VIHALS Motor Side Wire Holder (Autodesk Fusion 360 design; units mm, degrees)
Autodesk Fusion 360 part; units mm, degrees
sketch "Sketch1" plane through (0, 0, 0) normal (0, 0, 1) x (1, 0, 0)
  line L0 (-12.5, 10) -> (12.5, 10)
  line L1 (12.5, 10) -> (12.5, -10)
  line L2 (12.5, -10) -> (-12.5, -10)
  line L3 (-12.5, -10) -> (-12.5, 10)
  dimension "d1" = 25
  dimension "d2" = 12.5
  dimension "d3" = 20
  dimension "d4" = 10
  constraint horizontal L0
  constraint vertical L1
  constraint horizontal L2
  constraint vertical L3
  measures "d1" distance of L1 L3
  measures "d2" distance of origin L1
  measures "d3" distance of L0 L2
  measures "d4" distance of origin L0
extrude "Extrude1" add sketch "Sketch1" along normal blind 2
sketch "Sketch2" plane through (0, 0, 2) normal (0, 0, 1) x (-1, 0, 0)
  line L0 (12.5, 10) -> (-12.5, 10)
  line L1 (-12.5, 10) -> (-12.5, -10)
  line L2 (-12.5, -10) -> (12.5, -10)
  line L3 (12.5, -10) -> (12.5, 10)
  line L4 (12.5, 10) -> (14.5, 10)
  line L5 (14.5, 10) -> (14.5, -10)
  line L6 (14.5, -10) -> (12.5, -10)
  line L7 (12.5, -10) -> (12.5, 10)
  dimension "d7" = 2
  constraint horizontal L4
  constraint vertical L5
  constraint horizontal L6
  constraint vertical L7
  constraint coincident L0.start L3.end
  constraint horizontal L1.end L5.end
  measures "d7" distance of L5 L7
extrude "Extrude2" add sketch "Sketch2" along normal blind -2 and the other way blind -20 contours L3 L4 L5 L6 L7
sketch "Sketch3" plane through (0, 0, 22) normal (0, 0, 1) x (-1, 0, 0)
  line L0 (12.5, -10) -> (14.5, -10)
  line L1 (14.5, -10) -> (14.5, 10)
  line L2 (14.5, 10) -> (12.5, 10)
  line L3 (12.5, 10) -> (12.5, -10)
  line L4 (14.5, -10) -> (-12.5, -10)
  line L5 (-12.5, -10) -> (-12.5, 10)
  line L6 (-12.5, 10) -> (14.5, 10)
  line L7 (14.5, 10) -> (14.5, -10)
  point P0 (-12.5, 10)
  dimension "d12" = 27
  constraint horizontal L4
  constraint vertical L5
  constraint horizontal L6
  constraint vertical L7
  constraint coincident L0.end L1.start
  constraint horizontal L1.end P0
  measures "d12" distance of L5 L7
extrude "Extrude3" add sketch "Sketch3" along normal blind 2
ref_plane "WorkPlane1" through (0, 0, 23) normal (1, 0, 0) x (0, 1, 0)
sketch "Sketch8" plane through (0, 0, 0) normal (1, 0, 0) x (0, 1, 0)
  line L0 (-1.25, 37.553) -> (1.25, 37.553)
  line L1 (-9.7103, 24) -> (10, 24)
  circle A0 centre (-1.25, 32) radius 5
  circle A1 centre (1.25, 32) radius 5
  line L2 (1.25, 37.553) -> (1.25, 32)
  circle A2 centre (1.25, 32) radius 3
  line L3 (1.25, 32) -> (1.25, 24)
  circle A3 centre (-1.25, 32) radius 3
  line L4 (-1.25, 32) -> (-1.25, 24)
  line L5 (-1.25, 32) -> (-1.25, 37.553)
  line L6 (10, 24) -> (-10, 24)
  line L7 (-10, 24) -> (-10, 29)
  line L8 (-10, 29) -> (10, 29)
  line L9 (10, 29) -> (10, 24)
  point P0 (-9.7103, 23.053)
  point P1 (0, 22)
  point P2 (10, 23.053)
  point P3 (10, 24)
  point P4 (-10, 24)
  dimension "d73" = 10
  dimension "d74" = 10
  dimension "d75" = 10
  dimension "d76" = 2.5
  dimension "d77" = 1.25
  dimension "d78" = 6
  dimension "d79" = 6
  dimension "d80" = 2
  dimension "d93" = 3
  constraint horizontal A0.centre A1.centre
  constraint concentric A0 A3
  constraint concentric A1 A2
  constraint horizontal L1
  constraint coincident A0.centre A3.centre
  constraint coincident L4.end L1
  constraint perpendicular L1 L4
  constraint coincident A1.centre L2.end
  constraint coincident L3.end L1
  constraint perpendicular L1 L3
  constraint parallel L3 L5
  constraint perpendicular L0 L5
  constraint perpendicular L0 L2
  constraint vertical P0 L1.start
  constraint vertical P3 P2
  constraint vertical origin P1
  constraint coincident P3 L1.end
  constraint horizontal L6
  constraint vertical L7
  constraint horizontal L8
  constraint vertical L9
  constraint vertical L7.end P4
  measures "d73" diameter of A0
  measures "d74" diameter of A1
  measures "d75" vertical distance of A0.centre P1
  measures "d76" distance of A0.centre A1.centre
  measures "d77" horizontal distance of A1.centre P1
  measures "d78" diameter of A3
  measures "d79" diameter of A2
  measures "d80" distance of P1 L1
  measures "d93" distance of A0.centre L8
extrude "Extrude11" add 1 faces at (-4.1667, 3.3333, 2) along direction (0, 0, 1) blind 0.25
extrude "Extrude12" cut 1 faces at (-5.5, -3.3333, 0) along direction (0, 0, 1) blind 0.25
extrude "Extrude13" add sketch "Sketch8" along normal mid plane 3 contours A0 A1 A3 L5 L8 | A0 A1 L2 A2 L8 | A0 A1 L4 L8 | L1 A0 L4 L6 L7 L8 | A1 A3 L5 | A0 L2 A2 | A0 A1 L4 | L1 A0 A1 L3 L4 L6 | A1 L4 L8 | A1 A3 L8 | L1 A1 L3 L6 L8 L9 | A0 A1 L3 L8 | A0 A1 L3 L4 L8 | A0 A1 L3 | A0 A2 L8 | A0 L3 L8
fillet "Fillet13" radius 50 2 edges at (0, -5.25, 29) (0, 5.25, 29)
fillet "Fillet13" radius 1 2 edges at (0, -1.25, 37) (0, 1.25, 37)
chamfer "Chamfer1" distance 3 angle 45 2 edges at (1.5, 0, 24) (-1.5, 0, 24)
